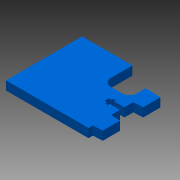
# Autodesk Inventor part: boardCaseBack
Saved by Autodesk Inventor 2013 (Build 170138000, 138)
## iProperties
Created: 2015-01-14
Part Number: boardCaseBack
Material: Generic
Document SubType Name: Modeling
Designer: dzban
Density: 1 g/cm^3
Author: dzban
Autodesk Inventor part; units mm, degrees
ref_plane "YZ Plane" through (0, 0, 0) normal (1, 0, 0) x (0, 1, 0)
ref_plane "XZ Plane" through (0, 0, 0) normal (0, 1, 0) x (-1, 0, 0)
ref_plane "XY Plane" through (0, 0, 0) normal (0, 0, 1) x (1, 0, 0)
sketch "Sketch1" plane through (0, 0, 0) normal (0, 0, 1) x (1, 0, 0)
  line L0 (0, 43) -> (-4, 43)
  line L1 (-4, 43) -> (-4, 37)
  arc A0 (-9, 32) -> (-4, 37) centre (-9, 37) ccw
  line L2 (-9, 32) -> (-17, 32)
  arc A1 (-22, 37) -> (-17, 32) centre (-17, 37) ccw
  line L3 (-22, 37) -> (-22, 52)
  line L4 (-22, 52) -> (-56.4, 52)
  line L5 (-56.4, 52) -> (-56.4, 0)
  line L6 (-56.4, 0) -> (0, 0)
  line L7 (0, 0) -> (0, 3)
  line L8 (0, 3) -> (6.4, 3.3)
  line L9 (6.4, 3.3) -> (6.4, 15.1)
  line L10 (6.4, 15.1) -> (0, 15.4)
  line L11 (0, 15.4) -> (0, 21.5)
  line L12 (0, 21.5) -> (-7, 21.5)
  line L13 (-7, 21.5) -> (-7, 20.25)
  line L14 (-7, 20.25) -> (-8.8, 20.25)
  line L15 (-8.8, 20.25) -> (-8.8, 21.5)
  line L16 (-8.8, 21.5) -> (-10.6, 21.5)
  line L17 (-10.6, 21.5) -> (-10.6, 24.5)
  line L18 (-10.6, 24.5) -> (-8.8, 24.5)
  line L19 (-8.8, 24.5) -> (-8.8, 25.75)
  line L20 (-8.8, 25.75) -> (-7, 25.75)
  line L21 (-7, 25.75) -> (-7, 24.5)
  line L22 (-7, 24.5) -> (0, 24.5)
  line L23 (0, 24.5) -> (0, 30.6)
  line L24 (0, 30.6) -> (6.4, 30.9)
  line L25 (6.4, 30.9) -> (6.4, 42.7)
  line L26 (6.4, 42.7) -> (0, 43)
  constraints: 54 end point, 4 point on circle, 2 centre point
extrude "Extrusion1" add sketch "Sketch1" along normal blind 6
body "Solid1"
